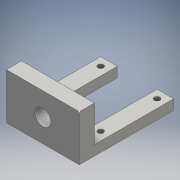
# Autodesk Inventor part: adapter
Saved by Autodesk Inventor 2016 (Build 200138000, 138)
## iProperties
Created: 2016-02-08
Part Number: adapter
Material: Generic
Document SubType Name: Modeling
Designer: Vervaeke-Lab
Density: 1 g/cm^3
Appearance: Default
Author: Vervaeke-Lab
Autodesk Inventor part; units mm, degrees
ref_plane "YZ Plane" through (0, 0, 0) normal (1, 0, 0) x (0, 1, 0)
ref_plane "XZ Plane" through (0, 0, 0) normal (0, 1, 0) x (-1, 0, 0)
ref_plane "XY Plane" through (0, 0, 0) normal (0, 0, 1) x (1, 0, 0)
sketch "Sketch1" plane through (0, 0, 0) normal (0, 1, 0) x (-1, 0, 0)
  line L0 (0, 0) -> (29, 0)
  line L1 (29, 0) -> (29, 18.3)
  line L2 (29, 18.3) -> (0, 18.3)
  line L3 (0, 18.3) -> (0, 0)
  dimension "d0" = 29
  dimension "d1" = 18.3
  constraints: 8 end point, 2 parallel, 1 horizontal, 1 perpendicular
  measures "d0" distance of L2.end L1.end
  measures "d1" distance of L1.end L0.end
extrude "Extrusion1" add sketch "Sketch1" along normal blind 6
sketch "Sketch2" plane through (0, 6, 0) normal (0, 1, 0) x (1, 0, 0)
  line L0 (0, 0) -> (-29, 0) projected
  line L1 (0, 0) -> (-6.6, 0)
  line L2 (-6.6, 0) -> (-6.6, -4)
  line L3 (-6.6, -4) -> (0, -4)
  line L4 (0, -4) -> (0, 0)
  dimension "d4" = 6.6
  dimension "d5" = 4
  constraints: 8 end point, 2 parallel, 1 horizontal, 1 perpendicular
  measures "d4" distance of L3.end L2.end
  measures "d5" distance of L2.end L1.end
extrude "Extrusion2" add sketch "Sketch2" along normal blind 31.5
sketch "Sketch3" plane through (0, 6, 0) normal (0, 1, 0) x (1, 0, 0)
  line L0 (-6.6, 0) -> (-29, 0) projected
  line L1 (-29, 0) -> (-22.4, 0)
  line L2 (-22.4, 0) -> (-22.4, -4)
  line L3 (-22.4, -4) -> (-29, -4)
  line L4 (-29, -4) -> (-29, 0)
  point P0 (0, 0)
  dimension "d8" = 6.6
  dimension "d9" = 4
  constraints: 8 end point, 2 parallel, 1 horizontal, 1 perpendicular
  measures "d8" distance of L2.end L3.end
  measures "d9" distance of L1.end L2.end
extrude "Extrusion3" add sketch "Sketch3" along normal blind 31.5
sketch "Sketch4" plane through (-6.6, 6, 4) normal (0, 0, 1) x (1, 0, 0)
  line L0 (-22.4, 0) -> (6.6, 0) projected
  point P0 (6.6, -6)
  point P1 (3.3, 5.8)
  point P2 (3.3, 5.8)
  point P3 (3.3, 28.2)
  point P4 (-19.1, 5.8)
  point P5 (-19.1, 28.2)
  dimension "d14" = 5.8
  dimension "d15" = 22.4
  dimension "d16" = 22.4
  dimension "d17" = 22.4
  dimension "d18" = 5.8
  constraints: 1 coincident
  measures "d14" distance from line of L0 point (3.3, 5.8)
  measures "d15" distance of point (3.3, 5.8) point (3.3, 28.2)
  measures "d16" distance of point (3.3, 28.2) point (-19.1, 28.2)
  measures "d17" distance of point (-19.1, 5.8) point (-19.1, 28.2)
  measures "d18" distance from line of L0 point (-19.1, 5.8)
hole "Hole1" at (-3.3, 11.8, 4) at (-3.3, 34.2, 4) at (-25.7, 11.8, 4) at (-25.7, 34.2, 4) direction (0, 0, -1) diameter 2.2 end through all
sketch "Sketch5" plane through (-29, 0, 18.3) normal (0, 0, 1) x (1, 0, 0)
  point P0 (29, 0)
sketch "Sketch6" plane through (0, 0, 0) normal (0, -1, 0) x (1, 0, 0)
  line L0 (-29, 18.3) -> (0, 18.3) projected
  point P0 (0, 0)
  point P1 (-14.5, 9.15)
  dimension "d26" = 9.15
  measures "d26" distance from line of L0 point (-14.5, 9.15)
hole "Hole2" at (-14.5, 0, 9.15) direction (0, 1, 0) diameter 6.35 end through all
body "Solid1"
